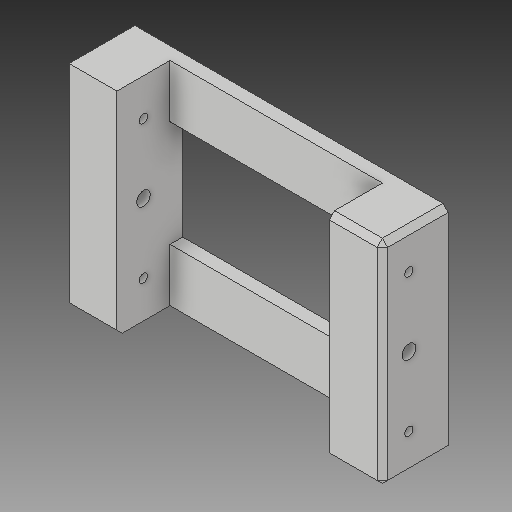
# Autodesk Inventor part: base box
Saved by Autodesk Inventor 2019 (Build 230136000, 136)
## iProperties
Created: 2020-02-16
Part Number: base box
Material: Generic
Document SubType Name: Modeling
Designer: JOHNWICK_58
Density: 1 g/cm^3
Appearance: Default
Author: JOHNWICK_58
Autodesk Inventor part; units mm, degrees
ref_plane "YZ Plane" through (0, 0, 0) normal (1, 0, 0) x (0, 1, 0)
ref_plane "XZ Plane" through (0, 0, 0) normal (0, 1, 0) x (-1, 0, 0)
ref_plane "XY Plane" through (0, 0, 0) normal (0, 0, 1) x (1, 0, 0)
sketch "Sketch1" plane through (0, 0, 0) normal (0, 0, 1) x (1, 0, 0)
  line L0 (0, 0) -> (300, 0)
  line L1 (300, 0) -> (300, 200)
  line L2 (300, 200) -> (0, 200)
  line L3 (0, 200) -> (0, 0)
  dimension "d0" = 300
  dimension "d1" = 200
  constraints: 8 end point, 2 parallel, 1 horizontal, 1 perpendicular
  measures "d0" distance of L2.end L1.end
  measures "d1" distance of L1.end L0.end
extrude "Extrusion1" add sketch "Sketch1" along normal blind 12
sketch "Sketch2" plane through (0, 0, 0) normal (0, 0, -1) x (-1, 0, 0)
  line L0 (-250, 150) -> (-50, 150)
  line L1 (-50, 150) -> (-50, 50)
  line L2 (-50, 50) -> (-250, 50)
  line L3 (-250, 50) -> (-250, 150)
  point P0 (0, 0)
  dimension "d4" = 200
  dimension "d5" = 100
  constraints: 8 end point, 2 parallel, 1 horizontal, 1 perpendicular
  measures "d4" distance of L1.end L2.end
  measures "d5" distance of L0.end L1.end
extrude "Extrusion2" cut sketch "Sketch2" against normal blind 19
sketch "Sketch3" plane through (0, 0, 12) normal (0, 0, 1) x (1, 0, 0)
  line L0 (0, 0) -> (300, 0) projected
  line L1 (300, 0) -> (250, 0)
  line L2 (250, 0) -> (250, 200)
  line L3 (250, 200) -> (300, 200)
  line L4 (300, 200) -> (300, 0)
  line L5 (0, 0) -> (50, 0)
  line L6 (50, 0) -> (50, 200)
  line L7 (50, 200) -> (0, 200)
  line L8 (0, 200) -> (0, 0)
  dimension "d8" = 50
  dimension "d9" = 200
  dimension "d10" = 50
  dimension "d11" = 200
  constraints: 16 end point, 4 parallel, 2 horizontal, 2 perpendicular
  measures "d8" distance of L2.end L3.end
  measures "d9" distance of L1.end L2.end
  measures "d10" distance of L7.end L6.end
  measures "d11" distance of L6.end L5.end
extrude "Extrusion3" add sketch "Sketch3" along normal blind 50
sketch "Sketch4" plane through (0, 0, 0) normal (-1, 0, 0) x (0, 0, 1)
  point P0 (0, 0)
sketch "Sketch5" plane through (0, 0, 0) normal (-1, 0, 0) x (0, 0, 1)
  circle A0 centre (37, 35) radius 4
  circle A1 centre (37, 100) radius 6.5
  circle A2 centre (37, 165) radius 4
  point P0 (0, 0)
  dimension "d14" = 8
  dimension "d15" = 13
  dimension "d16" = 8
  constraints: 3 centre point
  measures "d14" diameter of A0
  measures "d15" diameter of A1
  measures "d16" diameter of A2
extrude "Extrusion4" cut sketch "Sketch5" against normal blind 900
chamfer "Chamfer1" distance 5 angle 45 9 edges at (0, 100, 62) (0, 0, 31) (25, 0, 62) (275, 0, 62) (300, 100, 62) (275, 200, 62) (300, 200, 31) (0, 200, 31) (300, 0, 31)
body "Solid1"
